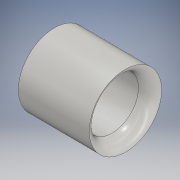
# Autodesk Inventor part: Deck_Bushing_Liner
Saved by Autodesk Inventor 2016 (Build 200138000, 138)
## iProperties
Created: 2016-05-07
Part Number: Deck_Bushing_Liner
Material: Stainless Steel
Document SubType Name: Modeling
Designer: agmle
Density: 8 g/cm^3
Appearance: Semi-Polished
Mass: 5.27092 g
Surface Area: 9.22476 cm^2
Volume: 0.658864 cm^3
Author: agmle
Autodesk Inventor part; units mm, degrees
ref_plane "YZ Plane" through (0, 0, 0) normal (1, 0, 0) x (0, 1, 0)
ref_plane "XZ Plane" through (0, 0, 0) normal (0, 1, 0) x (-1, 0, 0)
ref_plane "XY Plane" through (0, 0, 0) normal (0, 0, 1) x (1, 0, 0)
sketch "Sketch2" plane through (0, 0, 0) normal (0, 1, 0) x (-1, 0, 0)
  circle A0 centre (0, 0) radius 4.6
  circle A1 centre (0, 0) radius 6.3
  dimension "d14" = 9.2
  dimension "d15" = 1.7
  constraints: 2 centre point, 2 coincident
  measures "d14" diameter of A0
  measures "d15" radial gap between concentric circles of A1 A0
extrude "Extrusion1" add sketch "Sketch2" along normal blind 12.5
fillet "Fillet1" radius 2.5 2 edges at (4.6, 12.5, 0) (4.6, 0, 0)
body "Solid2"
